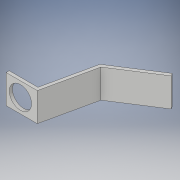
# Autodesk Inventor part: Spinner to Top
Saved by Autodesk Inventor 2017 (Build 210142000, 142)
## iProperties
Created: 2017-06-10
Part Number: Spinner to Top
Material: Generic
Document SubType Name: Modeling
Designer: Matthew
Density: 1 g/cm^3
Appearance: Default
Author: Matthew
Autodesk Inventor part; units mm, degrees
ref_plane "YZ Plane" through (0, 0, 0) normal (1, 0, 0) x (0, 1, 0)
ref_plane "XZ Plane" through (0, 0, 0) normal (0, 1, 0) x (-1, 0, 0)
ref_plane "XY Plane" through (0, 0, 0) normal (0, 0, 1) x (1, 0, 0)
sketch "Sketch1" plane through (0, 0, 0) normal (0, 1, 0) x (-1, 0, 0)
  line L0 (43.0137, 64.3915) -> (32.1817, 14.8739)
  line L1 (-10.5502, -12.5966) -> (-8.8333, -15.2673)
  line L2 (-8.8333, -15.2673) -> (35.0028, 12.913)
  line L3 (35.0028, 12.913) -> (46.1153, 63.713)
  line L4 (46.1153, 63.713) -> (43.0137, 64.3915)
  line L5 (-10.5502, -12.5966) -> (-10.5502, 12.913)
  line L6 (-10.5502, -12.5966) -> (32.1817, 14.8739)
  line L7 (46.1153, 63.713) -> (74.6903, 63.713)
  line L8 (74.6903, 63.713) -> (74.6903, 66.888)
  line L9 (74.6903, 66.888) -> (43.5598, 66.888)
  line L10 (43.0137, 64.3915) -> (43.5598, 66.888)
  point P0 (0, 0)
  dimension "d0" = 3.175
  dimension "d1" = 3.175
  dimension "d3" = 50.8
  dimension "d4" = 57.265
  dimension "d5" = 50.8
  dimension "d6" = 11.1125
  dimension "d7" = 28.575
  dimension "d8" = 3.175
  constraints: 22 end point, 4 perpendicular, 3 vertical, 1 collinear, 1 horizontal, 1 parallel, 1 other
  measures "d0" distance of L1.start L1.end
  measures "d1" distance of L3.end L0.start
  measures "d3" distance of L1.start L0.end
  measures "d4" angle of L5 L6
  measures "d5" vertical distance of L2.end L3.end
  measures "d6" horizontal distance of L2.end L3.end
  measures "d7" distance of L3.end L7.end
  measures "d8" distance of L7.end L8.end
extrude "Extrusion1" add sketch "Sketch1" along normal blind 28.575
sketch "Sketch2" plane through (-74.6903, 0, 66.888) normal (0, 0, 1) x (1, 0, 0)
  line L0 (28.575, 0) -> (0, 0) projected
  line L1 (0, 0) -> (0, 28.575) projected
  line L2 (28.575, 28.575) -> (0, 28.575) projected
  line L3 (28.575, 0) -> (28.575, 28.575) projected
  line L4 (28.575, 28.575) -> (0, 28.575) projected
  line L5 (0, 0) -> (0, 28.575) projected
  circle A0 centre (14.2875, 14.2875) radius 11.1125
  point P0 (74.6903, 0)
  point P1 (14.2875, 28.575)
  point P2 (0, 14.2875)
  dimension "d11" = 22.225
  constraints: 2 midpoint, 1 centre point
  measures "d11" diameter of A0
extrude "Extrusion2" cut sketch "Sketch2" against normal blind 28.575 contours A0
body "Solid1"
